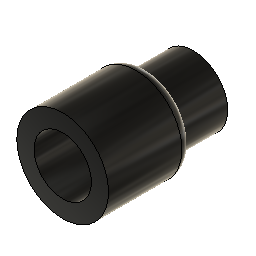
PropellerAdaprter5ToBearing6 v2 (Autodesk Fusion 360 design; units mm, degrees)
Autodesk Fusion 360 part; units mm, degrees
sketch "Sketch1" plane through (0, 0, 0) normal (0, 1, 0) x (1, 0, 0)
  circle A0 centre (0, 0) radius 2.5
  circle A1 centre (0, 0) radius 4
  dimension "d1" = 5
  dimension "d2" = 8
  constraint coincident A0.centre A1.centre
  measures "d1" diameter of A0
  measures "d2" diameter of A1
extrude "Extrude1" add sketch "Sketch1" along normal blind 7.4
sketch "Sketch2" plane through (0, 7.4, 0) normal (0, 1, 0) x (-1, 0, 0)
  circle A0 centre (0, 0) radius 2.5
  circle A1 centre (0, 0) radius 4
  circle A2 centre (0, 0) radius 3
  dimension "d5" = 6
  constraint coincident A0.centre A1.centre
  measures "d5" diameter of A2
extrude "Extrude2" add sketch "Sketch2" along normal blind 4 contours A2
fillet "Fillet1" radius 1 1 edges at (-3.7293, 7.4, 1.4465)
